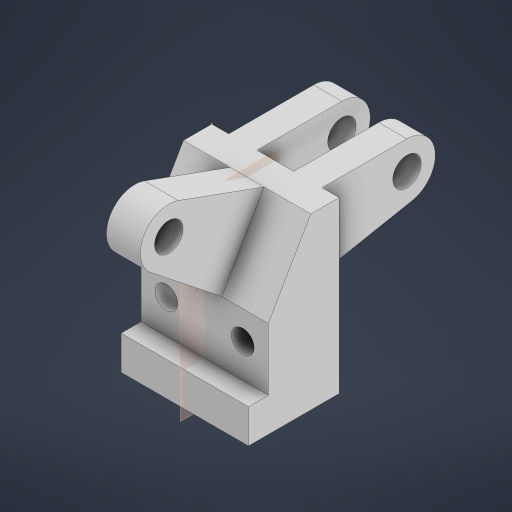
# Autodesk Inventor part: Część18
Saved by Autodesk Inventor 2023 (Build 270158000, 158)
## iProperties
Created: 2023-05-08
Part Number: Część18
Material: Ogólny
Document SubType Name: Modeling
Designer: Adam
Density: 1 g/cm^3
Appearance: Domyślna
Author: Adam
Autodesk Inventor part; units mm, degrees
ref_plane "YZ Plane" through (0, 0, 0) normal (1, 0, 0) x (0, 1, 0)
ref_plane "XZ Plane" through (0, 0, 0) normal (0, 1, 0) x (-1, 0, 0)
ref_plane "XY Plane" through (0, 0, 0) normal (0, 0, 1) x (1, 0, 0)
sketch "Szkic1" plane through (0, 0, 0) normal (0, 1, 0) x (-1, 0, 0)
  line L0 (0, 0) -> (-45, 0)
  line L1 (-45, 0) -> (-45, 32)
  line L2 (-45, 32) -> (0, 32)
  line L3 (0, 32) -> (0, 0)
  dimension "d0" = 45
  dimension "d1" = 32
  constraints: 8 end point, 2 parallel, 1 horizontal, 1 perpendicular
  measures "d0" distance of L1.end L2.end
  measures "d1" distance of L0.end L1.end
extrude "Wyciągnięcie proste1" add sketch "Szkic1" along normal blind 12
sketch "Szkic2" plane through (0, 12, 0) normal (0, 1, 0) x (1, 0, 0)
  line L0 (45, 0) -> (0, 0) projected
  line L1 (45, -32) -> (45, 0) projected
  line L2 (0, 0) -> (45, 0)
  line L3 (45, 0) -> (45, -25)
  line L4 (45, -25) -> (0, -25)
  line L5 (0, -25) -> (0, 0)
  constraints: 8 end point, 2 parallel, 1 horizontal, 1 perpendicular, 1 point on line
extrude "Wyciągnięcie proste2" add sketch "Szkic2" along normal blind 48
sketch "Szkic3" plane through (0, 12, 25) normal (0, 0, 1) x (1, 0, 0)
  point P0 (0, -12)
  point P1 (9, 12)
  point P2 (36, 12)
hole "Otwór1" at (9, 24, 25) at (36, 24, 25) direction (0, 0, -1) diameter 8 end through all
chamfer "Faza1" distance 26 angle 30 1 edges at (22.5, 60, 25) measured on face at (26.3804, 49.1806, 25)
sketch "Szkic4" plane through (0, 60, 0) normal (0, 1, 0) x (1, 0, 0)
  point P0 (0, 0)
ref_plane "Płaszczyzna konstrukcyjna1" through (22.5, 0, 32) normal (1, 0, 0) x (0, 0, -1)
sketch "Szkic5" plane through (22.5, 0, 32) normal (1, 0, 0) x (0, 0, -1)
  circle A0 centre (-11.7045, 61.6029) radius 10
  line L0 (7, 34) -> (22.0111, 60) projected
  line L1 (22.0111, 60) -> (-8.2916, 71.0025)
  line L2 (7, 12) -> (7, 34) projected
  line L3 (7, 34) -> (-17.9194, 53.7687)
  point P0 (32, 0)
  dimension "d16" = 20
  dimension "d17" = 30
  constraints: 4 end point, 2 point on circle, 2 tangent, 1 centre point
  measures "d16" diameter of A0
  measures "d17" distance from line of L0 A0.centre
extrude "Wyciągnięcie proste3" add sketch "Szkic5" along normal mid plane 12
sketch "Szkic6" plane through (28.5, 0, 32) normal (1, 0, 0) x (0, 0, -1)
  arc A0 (-8.2916, 71.0025) -> (-17.9194, 53.7687) centre (-11.7045, 61.6029) ccw projected
  point P0 (32, 0)
  constraints: 1 coincident
hole "Otwór2" at (28.5, 61.6029, 43.7045) direction (-1, 0, 0) diameter 10 end through all
sketch "Szkic7" plane through (28.5, 0, 32) normal (1, 0, 0) x (0, 0, -1)
  point P0 (32, 0)
sketch "Szkic8" plane through (22.5, 0, 32) normal (1, 0, 0) x (0, 0, -1)
  circle A0 centre (62, 50) radius 10
  line L0 (32, 0) -> (32, 60) projected
  line L1 (32, 60) -> (62, 60)
  line L2 (32, 34) -> (63.9026, 40.1827)
  dimension "d27" = 20
  dimension "d28" = 30
  dimension "d30" = 26
  constraints: 4 end point, 2 horizontal, 1 point on line, 4 other
  measures "d28" distance from line of point (62, 50) L0
  measures "d30" distance from line of L2.start L1
extrude "Wyciągnięcie proste4" add sketch "Szkic8" along normal mid plane 33
sketch "Szkic9" plane through (22.5, 0, 32) normal (1, 0, 0) x (0, 0, -1)
  arc A0 (63.9026, 40.1827) -> (62, 60) centre (62, 50) ccw projected
  line L0 (32, 60) -> (22.0111, 60) projected
  line L1 (62, 60) -> (32, 60)
  line L2 (32, 60) -> (32, 34)
  line L3 (32, 0) -> (32, 60) projected
  line L4 (32, 34) -> (63.9026, 40.1827) projected
  line L5 (62, 60) -> (32, 60) projected
  arc A1 (63.9026, 40.1827) -> (62, 60) centre (62.5165, 50.0496) ccw
  constraints: 4 end point, 2 point on circle, 1 centre point, 1 collinear, 1 point on line
extrude "Wyciągnięcie proste5" cut sketch "Szkic9" along normal mid plane 13 contours L4 L2 L1 A0
sketch "Szkic10" plane through (39, 0, 32) normal (1, 0, 0) x (0, 0, -1)
  point P0 (32, 0)
sketch "Szkic11" plane through (39, 0, 32) normal (1, 0, 0) x (0, 0, -1)
  arc A0 (63.9026, 40.1827) -> (62, 60) centre (62, 50) ccw projected
  point P0 (32, 0)
  constraints: 1 coincident
hole "Otwór3" at (39, 50, -30) direction (-1, 0, 0) diameter 10 end through all
